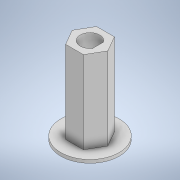
# Autodesk Inventor part: pressfit
Saved by Autodesk Inventor 2020 (Build 240168000, 168)
## iProperties
Created: 2019-12-28
Part Number: pressfit
Material: Generic
Document SubType Name: Modeling
Designer: xj82b
Density: 1 g/cm^3
Appearance: Default
Author: xj82b
Autodesk Inventor part; units mm, degrees
ref_plane "YZ Plane" through (0, 0, 0) normal (1, 0, 0) x (0, 1, 0)
ref_plane "XZ Plane" through (0, 0, 0) normal (0, 1, 0) x (-1, 0, 0)
ref_plane "XY Plane" through (0, 0, 0) normal (0, 0, 1) x (1, 0, 0)
sketch "Sketch1" plane through (0, 0, 0) normal (0, 1, 0) x (-1, 0, 0)
  line L0 (-11.5624, -8.1191) -> (-8.8128, -12.8816)
  line L1 (-8.8128, -12.8816) -> (-11.5624, -17.6441)
  line L2 (-11.5624, -17.6441) -> (-17.0617, -17.6441)
  line L3 (-17.0617, -17.6441) -> (-19.8113, -12.8816)
  line L4 (-19.8113, -12.8816) -> (-17.0617, -8.1191)
  line L5 (-17.0617, -8.1191) -> (-11.5624, -8.1191)
  line L6 (0, 0) -> (-27.888, 0) construction
  arc A0 (-16.812, -14.54) -> (-16.812, -11.2233) centre (-14.312, -12.8816) ccw
  line L7 (-16.812, -14.54) -> (-16.812, -11.2233)
  dimension "d0" = 9.525
  dimension "d1" = 6
  dimension "d2" = 5.5
  constraints: 16 end point, 2 point on circle, 1 centre point, 1 coincident, 1 horizontal, 1 parallel, 1 vertical, 13 other
  measures "d0" distance between parallel lines of L5 L2
  measures "d1" diameter of A0
extrude "Extrusion1" add sketch "Sketch1" along normal blind 25.4
sketch "Sketch2" plane through (0, 0, 0) normal (0, -1, 0) x (1, 0, 0)
  circle A0 centre (14.312, -12.8816) radius 9
  arc A1 (16.812, -11.2233) -> (16.812, -14.54) centre (14.312, -12.8816) ccw projected
  arc A2 (16.812, -11.2233) -> (16.812, -14.54) centre (14.312, -12.8816) ccw
  line L0 (16.812, -11.2233) -> (16.812, -14.54)
  point P0 (0, 0)
  point P1 (16.812, -14.54)
  dimension "d5" = 18
  dimension "d6" = 6
  dimension "d7" = 5.5
  constraints: 2 centre point, 2 concentric, 2 end point, 2 point on circle, 1 vertical
  measures "d5" diameter of A0
  measures "d6" diameter of A2
extrude "Extrusion2" add sketch "Sketch2" along normal blind 1
body "Solid1"
